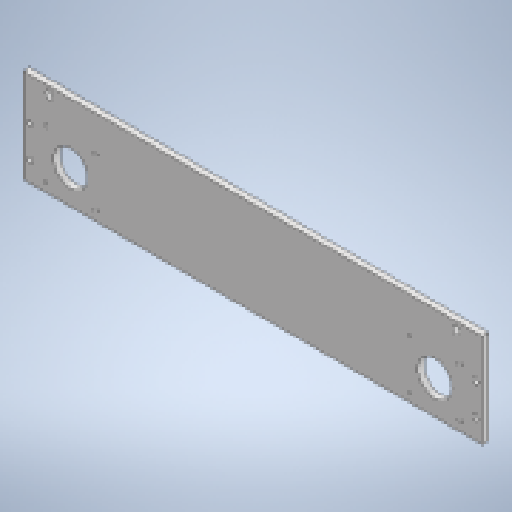
# Autodesk Inventor part: креп_мотора
Saved by Autodesk Inventor 2023.1 (Build 271208000, 208)
## iProperties
Created: 2025-12-22
Part Number: креп_мотора
Material: Типовые
Document SubType Name: Modeling
Designer: DELL
Density: 1 g/cm^3
Appearance: По умолчанию
Author: DELL
Autodesk Inventor part; units mm, degrees
ref_plane "YZ Plane" through (0, 0, 0) normal (1, 0, 0) x (0, 1, 0)
ref_plane "XZ Plane" through (0, 0, 0) normal (0, 1, 0) x (-1, 0, 0)
ref_plane "XY Plane" through (0, 0, 0) normal (0, 0, 1) x (1, 0, 0)
sketch "Эскиз1" plane through (0, 0, 0) normal (0, 0, 1) x (1, 0, 0)
  circle A0 centre (-15.5, -15.5) radius 1.25 projected
  circle A1 centre (-15.5, 15.5) radius 1.25 projected
  circle A2 centre (15.5, 15.5) radius 1.25 projected
  circle A3 centre (15.5, -15.5) radius 1.25 projected
  circle A4 centre (25.65, -8.65) radius 1.75 projected
  circle A5 centre (25.65, 11.35) radius 1.75 projected
  circle A6 centre (0, 0) radius 11 projected
  line L0 (29.95, -21.15) -> (21.35, -21.15) construction
  line L1 (-21.15, 17.0257) -> (-21.15, -17.0257) construction
  line L2 (17.0257, 21.15) -> (-17.0257, 21.15) construction
  line L3 (29.95, -21.15) -> (-260.45, -21.15)
  line L4 (-260.45, -21.15) -> (-260.45, 38.15)
  line L5 (-260.45, 38.15) -> (29.95, 38.15)
  line L6 (29.95, 38.15) -> (29.95, -21.15)
  circle A7 centre (25.65, 11.35) radius 4.5 construction
  line L7 (31.65, 11.35) -> (31.65, 31.2297) construction
  line L8 (19.65, 11.35) -> (19.65, 31.2297) construction
  circle A8 centre (13.65, 33.15) radius 2.5
  circle A9 centre (13.65, 33.15) radius 6 construction
  circle A10 centre (13.65, 33.15) radius 9 construction
  line L9 (-260.45, -21.15) -> (-260.45, 278.85) projected
  line L10 (-115.25, -21.15) -> (-115.25, 21.2899) construction
  circle A11 centre (-215, -15.5) radius 1.25
  circle A12 centre (-215, 15.5) radius 1.25
  circle A13 centre (-246, 15.5) radius 1.25
  circle A14 centre (-246, -15.5) radius 1.25
  circle A15 centre (-256.15, -8.65) radius 1.75
  circle A16 centre (-256.15, 11.35) radius 1.75
  circle A17 centre (-230.5, 0) radius 11
  line L11 (-209.35, 17.0257) -> (-209.35, -17.0257) construction
  line L12 (-247.5257, 21.15) -> (-213.4743, 21.15) construction
  circle A18 centre (-256.15, 11.35) radius 4.5 construction
  line L13 (-250.15, 11.35) -> (-250.15, 31.2297) construction
  circle A19 centre (-244.15, 33.15) radius 2.5
  circle A20 centre (-244.15, 33.15) radius 6 construction
  circle A21 centre (-244.15, 33.15) radius 9 construction
  point P0 (0, 0)
  point P1 (-260.45, 8.5)
  point P2 (-230.5, 0)
  dimension "d3" = 5
  dimension "d4" = 12
  dimension "d5" = 18
  dimension "d6" = 12
  dimension "d7" = 5
  constraints: 20 end point, 18 symmetric about line, 14 centre point, 4 coincident, 3 vertical, 2 midpoint, 2 parallel, 1 horizontal, 1 perpendicular, 1 point on line, 1 tangent, 11 other
  measures "d3" diameter of A8
  measures "d4" diameter of A9
  measures "d5" diameter of A10
  measures "d6" distance from line of L2 A8.centre
  measures "d7" distance from line of L5 A8.centre
extrude "Выдавливание1" add sketch "Эскиз1" along normal blind 6
